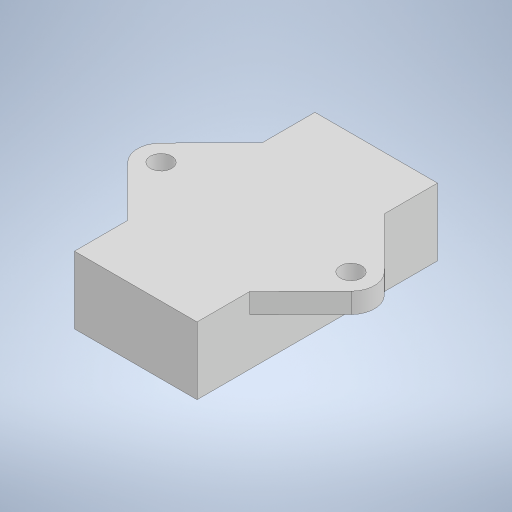
# Autodesk Inventor part: креп_опт
Saved by Autodesk Inventor 2023.1 (Build 271208000, 208)
## iProperties
Created: 2025-12-30
Part Number: креп_опт
Material: Типовые
Document SubType Name: Modeling
Designer: DELL
Density: 1 g/cm^3
Appearance: По умолчанию
Author: DELL
Autodesk Inventor part; units mm, degrees
ref_plane "YZ Plane" through (0, 0, 0) normal (1, 0, 0) x (0, 1, 0)
ref_plane "XZ Plane" through (0, 0, 0) normal (0, 1, 0) x (-1, 0, 0)
ref_plane "XY Plane" through (0, 0, 0) normal (0, 0, 1) x (1, 0, 0)
sketch "Эскиз1" plane through (0, 0, 0) normal (0, 1, 0) x (-1, 0, 0)
  line L0 (7.1, -15.85) -> (-7.1, -15.85)
  line L1 (-7.1, -15.85) -> (-7.1, 15.85)
  line L2 (-7.1, 15.85) -> (7.1, 15.85)
  line L3 (7.1, 15.85) -> (7.1, -15.85)
  line L4 (7.1, -15.85) -> (-7.1, 15.85) construction
  line L5 (-7.1, -15.85) -> (7.1, 15.85) construction
  line L6 (9.1, -17.85) -> (-9.1, -17.85)
  line L7 (-9.1, -17.85) -> (-9.1, 17.85)
  line L8 (-9.1, 17.85) -> (9.1, 17.85)
  line L9 (9.1, 17.85) -> (9.1, -17.85)
  point P0 (0, 0)
  dimension "d0" = 14.2
  dimension "d1" = 31.7
  dimension "d2" = 2
  constraints: 20 end point, 4 parallel, 2 midpoint, 2 perpendicular, 1 horizontal, 3 other
  measures "d0" distance of L1.end L2.end
  measures "d1" distance of L2.end L0.start
  measures "d2" distance between parallel lines of L3 L9
extrude "Выдавливание1" add sketch "Эскиз1" along normal blind 7
sketch "Эскиз2" plane through (0, 7, 0) normal (0, 1, 0) x (1, 0, 0)
  line L0 (-9.1, 17.85) -> (-9.1, -17.85) projected
  line L1 (-9.1, -17.85) -> (9.1, -17.85) projected
  line L2 (9.1, -17.85) -> (9.1, 17.85) projected
  line L3 (9.1, 17.85) -> (-9.1, 17.85) projected
  point P0 (0, 0)
extrude "Выдавливание2" add sketch "Эскиз2" along normal blind 3
sketch "Эскиз4" plane through (9.1, 0, -17.85) normal (0, 0, -1) x (-1, 0, 0)
  line L0 (0, 0) -> (0, 10) construction
  line L1 (0, 0) -> (0, 10) construction
  line L2 (0, 0) -> (18.2, 0) construction
  line L3 (18.2, 0) -> (18.2, 10) construction
  line L4 (18.2, 0) -> (18.2, 10) construction
  line L5 (0, 0) -> (0, 10) projected
  line L6 (0, 0) -> (0, 10)
  line L7 (18.2, 0) -> (0, 0) projected
  line L8 (0, 0) -> (18.2, 0)
  line L9 (18.2, 0) -> (18.2, 10)
  line L10 (5.972, 10) -> (0, 10)
  line L11 (0, 10) -> (18.2, 10)
  line L12 (0, 0) -> (0, 10) projected
  line L13 (0, 10) -> (0, 7)
  line L14 (2, 0) -> (2, 7)
  line L15 (2, 7) -> (16.2, 7)
  line L16 (16.2, 7) -> (16.2, 0)
  point P0 (9.1, 0)
  point P1 (18.2, 7)
  point P2 (0, 5)
  point P3 (18.2, 5)
  point P4 (16.2, 0)
  dimension "d15" = 2
  dimension "d16" = 2
  constraints: 18 end point, 4 perpendicular, 3 collinear, 2 midpoint, 2 point on line
  measures "d15" distance from line of point (0, 5) L14
  measures "d16" distance from line of point (18.2, 5) L16
extrude "Выдавливание4" cut sketch "Эскиз4" against normal blind 3 contours L14 L15 L16 L7
sketch "Эскиз5" plane through (0, 10, 0) normal (0, 1, 0) x (1, 0, 0)
  circle A0 centre (14.1, 0) radius 1.6
  circle A1 centre (-14.1, 0) radius 1.6
  line L0 (-9.1, 17.85) -> (-9.1, -17.85) projected
  line L1 (9.1, -17.85) -> (9.1, 17.85) projected
  arc A2 (16.5831, -2.4666) -> (16.5831, 2.4666) centre (14.1, 0) ccw
  arc A3 (-16.5831, 2.4666) -> (-16.5831, -2.4666) centre (-14.1, 0) ccw
  line L2 (9.1, -10) -> (16.5831, -2.4666)
  line L3 (16.5831, 2.4666) -> (9.1, 10)
  line L4 (9.1, -17.85) -> (9.1, 17.85) projected
  line L5 (-16.5831, -2.4666) -> (-9.1, -10)
  line L6 (-16.5831, 2.4666) -> (-9.1, 10)
  point P0 (0, 0)
  point P1 (9.1, 0)
  point P2 (9.1, 0)
  point P3 (-9.1, 0)
  point P4 (-9.1, 0)
  dimension "d20" = 3.2
  dimension "d21" = 3.2
  dimension "d22" = 5
  dimension "d23" = 5
  dimension "d24" = 7
  dimension "d25" = 7
  dimension "d26" = 10
  dimension "d27" = 10
  dimension "d28" = 10
  dimension "d29" = 10
  constraints: 8 end point, 4 centre point, 4 midpoint, 4 point on circle, 4 point on line, 4 tangent, 2 coincident
  measures "d20" diameter of A0
  measures "d21" diameter of A1
  measures "d22" distance from line of L0 A1.centre
  measures "d23" distance from line of A0.centre L1
  measures "d24" diameter of A2
  measures "d25" diameter of A3
  measures "d26" distance of point (9.1, 0) L2.start
  measures "d27" distance of L3.end point (9.1, 0)
  measures "d28" distance of point (-9.1, 0) L5.end
  measures "d29" distance of point (-9.1, 0) L6.end
extrude "Выдавливание5" add sketch "Эскиз5" against normal blind 3
